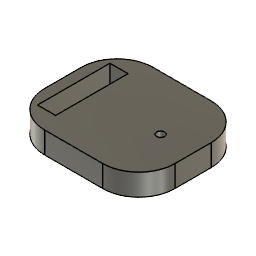
Vtol main body rib (Autodesk Fusion 360 design; units mm, degrees)
part number: 2026-06-17-15-36-35-159
Autodesk Fusion 360 part; units mm, degrees
sketch "Sketch1" plane through (0, 0, 0) normal (0, 0, 1) x (1, 0, 0)
  line L0 (-40, -75) -> (40, -75)
  line L1 (90, -25) -> (90, 25)
  line L2 (40, 75) -> (-40, 75)
  line L3 (-90, 25) -> (-90, -25)
  line L4 (-90, -75) -> (90, 75) construction
  line L5 (90, -75) -> (-90, 75) construction
  arc A0 (40, -75) -> (90, -25) centre (40, -25) ccw
  arc A1 (90, 25) -> (40, 75) centre (40, 25) ccw
  arc A2 (-90, -25) -> (-40, -75) centre (-40, -25) ccw
  arc A3 (-40, 75) -> (-90, 25) centre (-40, 25) ccw
  constraint horizontal L0
  constraint perpendicular L0 L1
  constraint parallel L0 L2
  constraint parallel L1 L3
  constraint coincident L4 origin
  constraint coincident L5 origin
  constraint coincident L5.start L1
  constraint coincident L5.start L0
  constraint tangent L1 A0
  constraint tangent L0 A0
  constraint coincident L4.end L1
  constraint coincident L4.end L2
  constraint tangent L1 A1
  constraint tangent L2 A1
  constraint coincident L4.start L0
  constraint coincident L4.start L3
  constraint tangent L0 A2
  constraint tangent L3 A2
  constraint coincident L5.end L2
  constraint coincident L5.end L3
  constraint tangent L2 A3
  constraint tangent L3 A3
extrude "Extrude1" add sketch "Sketch1" along normal blind 30
sketch "Sketch2" plane through (0, 0, 30) normal (0, 0, 1) x (-1, 0, 0)
  arc A0 (40, -75) -> (90, -25) centre (40, -25) ccw
  line L0 (90, -25) -> (90, 25)
  arc A1 (90, 25) -> (40, 75) centre (40, 25) ccw
  line L1 (40, 75) -> (-40, 75)
  arc A2 (-40, 75) -> (-90, 25) centre (-40, 25) ccw
  line L2 (-90, 25) -> (-90, -25)
  arc A3 (-90, -25) -> (-40, -75) centre (-40, -25) ccw
  line L3 (-40, -75) -> (40, -75)
  line L4 (35, 70) -> (-35, 70)
  line L5 (-85, 20) -> (-85, -20)
  line L6 (-35, -70) -> (35, -70)
  line L7 (85, -20) -> (85, 20)
  line L8 (85, 70) -> (-85, -70) construction
  line L9 (-85, 70) -> (85, -70) construction
  arc A4 (-35, 70) -> (-85, 20) centre (-35, 20) ccw
  arc A5 (-85, -20) -> (-35, -70) centre (-35, -20) ccw
  arc A6 (85, 20) -> (35, 70) centre (35, 20) ccw
  arc A7 (35, -70) -> (85, -20) centre (35, -20) ccw
  dimension "d9" = 140
  dimension "d10" = 170
  dimension "d11" = 50
  dimension "d12" = 50
  dimension "d13" = 50
  dimension "d14" = 50
  constraint horizontal L4
  constraint perpendicular L4 L5
  constraint parallel L4 L6
  constraint parallel L5 L7
  constraint coincident L8 origin
  constraint coincident L9 origin
  constraint coincident L9.start L5
  constraint coincident L9.start L4
  constraint tangent L5 A4
  constraint tangent L4 A4
  constraint coincident L8.end L5
  constraint coincident L8.end L6
  constraint tangent L5 A5
  constraint tangent L6 A5
  constraint coincident L8.start L4
  constraint coincident L8.start L7
  constraint tangent L4 A6
  constraint tangent L7 A6
  constraint coincident L9.end L6
  constraint coincident L9.end L7
  constraint tangent L6 A7
  constraint tangent L7 A7
  measures "d9" distance of L9.start L8.end
  measures "d10" distance of L8.end L9.end
  measures "d11" radius of A4
  measures "d12" radius of A5
  measures "d13" radius of A6
  measures "d14" radius of A7
extrude "Extrude2" cut sketch "Sketch2" against normal blind 10 contours L4 L5 L6 L7 A4 A5 A6 A7
sketch "Sketch3" plane through (0, 0, 0) normal (0, 0, -1) x (1, 0, 0)
  arc A0 (-90, -25) -> (-40, -75) centre (-40, -25) ccw
  line L0 (-40, -75) -> (40, -75)
  arc A1 (40, -75) -> (90, -25) centre (40, -25) ccw
  line L1 (90, -25) -> (90, 25)
  arc A2 (90, 25) -> (40, 75) centre (40, 25) ccw
  line L2 (40, 75) -> (-40, 75)
  arc A3 (-40, 75) -> (-90, 25) centre (-40, 25) ccw
  line L3 (-90, 25) -> (-90, -25)
  line L4 (-35, -70) -> (35, -70)
  line L5 (85, -20) -> (85, 20)
  line L6 (35, 70) -> (-35, 70)
  line L7 (-85, 20) -> (-85, -20)
  line L8 (-85, -70) -> (85, 70) construction
  line L9 (85, -70) -> (-85, 70) construction
  arc A4 (35, -70) -> (85, -20) centre (35, -20) ccw
  arc A5 (85, 20) -> (35, 70) centre (35, 20) ccw
  arc A6 (-85, -20) -> (-35, -70) centre (-35, -20) ccw
  arc A7 (-35, 70) -> (-85, 20) centre (-35, 20) ccw
  dimension "d17" = 140
  dimension "d18" = 170
  dimension "d19" = 50
  dimension "d20" = 50
  dimension "d21" = 50
  dimension "d22" = 50
  constraint horizontal L4
  constraint perpendicular L4 L5
  constraint parallel L4 L6
  constraint parallel L5 L7
  constraint coincident L8 origin
  constraint coincident L9 origin
  constraint coincident L9.start L5
  constraint coincident L9.start L4
  constraint tangent L5 A4
  constraint tangent L4 A4
  constraint coincident L8.end L5
  constraint coincident L8.end L6
  constraint tangent L5 A5
  constraint tangent L6 A5
  constraint coincident L8.start L4
  constraint coincident L8.start L7
  constraint tangent L4 A6
  constraint tangent L7 A6
  constraint coincident L9.end L6
  constraint coincident L9.end L7
  constraint tangent L6 A7
  constraint tangent L7 A7
  measures "d17" distance of L9.start L8.end
  measures "d18" distance of L8.end L9.end
  measures "d19" radius of A4
  measures "d20" radius of A5
  measures "d21" radius of A6
  measures "d22" radius of A7
extrude "Extrude3" cut sketch "Sketch3" against normal blind 10 contours L4 L5 L6 L7 A4 A5 A6 A7
sketch "Sketch4" plane through (0, 0, 10) normal (0, 0, -1) x (1, 0, 0)
  arc A0 (-35, 70) -> (-85, 20) centre (-35, 20) ccw
  line L0 (-85, 20) -> (-85, -20)
  arc A1 (-85, -20) -> (-35, -70) centre (-35, -20) ccw
  line L1 (-35, -70) -> (35, -70)
  arc A2 (35, -70) -> (85, -20) centre (35, -20) ccw
  line L2 (85, -20) -> (85, 20)
  arc A3 (85, 20) -> (35, 70) centre (35, 20) ccw
  line L3 (35, 70) -> (-35, 70)
  line L4 (90, 0) -> (45, 0)
  circle A4 centre (45, 0) radius 5.5
  dimension "d25" = 45
  dimension "d26" = 11
  constraint perpendicular L2 L4
  constraint coincident L4.end A4.centre
  measures "d25" distance of L4.start L4.end
  measures "d26" diameter of A4
extrude "Extrude4" cut sketch "Sketch4" against normal blind 10 contours A4
extrude "Extrude5" add 1 faces at (-26.8129, 30.2732, 20) along direction (0, 0, 1) blind 10
extrude "Extrude6" add 1 faces at (-26.8129, 30.2732, 10) along direction (0, 0, -1) blind 10
sketch "Sketch5" plane through (0, 0, 0) normal (0, 0, -1) x (1, 0, 0)
  circle A0 centre (45, 0) radius 5.5
  arc A1 (-90, -25) -> (-40, -75) centre (-40, -25) ccw
  line L0 (-40, -75) -> (40, -75)
  arc A2 (40, -75) -> (90, -25) centre (40, -25) ccw
  line L1 (90, -25) -> (90, 25)
  arc A3 (90, 25) -> (40, 75) centre (40, 25) ccw
  line L2 (40, 75) -> (-40, 75)
  arc A4 (-40, 75) -> (-90, 25) centre (-40, 25) ccw
  line L3 (-90, 25) -> (-90, -25)
  line L4 (-75, 50) -> (-50, 50)
  line L5 (-50, 50) -> (-50, -50)
  line L6 (-50, -50) -> (-75, -50)
  line L7 (-75, -50) -> (-75, 50)
  constraint horizontal L4
  constraint vertical L5
  constraint horizontal L6
  constraint vertical L7
extrude "Extrude7" cut sketch "Sketch5" against normal blind 65 contours L4 L5 L6 L7
